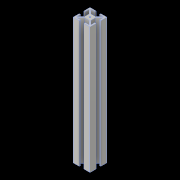
# Autodesk Inventor part: ProfileOne
Saved by Autodesk Inventor 2016 (Build 200138000, 138)
## iProperties
Created: 2017-01-21
Part Number: ProfileOne
Material: Generic
Document SubType Name: Modeling
Designer: Alexis Renderos
Density: 1 g/cm^3
Appearance: Aluminum - Flat
Author: Alexis Renderos
Autodesk Inventor part; units mm, degrees
ref_plane "YZ Plane" through (0, 0, 0) normal (1, 0, 0) x (0, 1, 0)
ref_plane "XZ Plane" through (0, 0, 0) normal (0, 1, 0) x (-1, 0, 0)
ref_plane "XY Plane" through (0, 0, 0) normal (0, 0, 1) x (1, 0, 0)
sketch "Sketch1" plane through (0, 0, 0) normal (0, 1, 0) x (-1, 0, 0)
  line L0 (0, -21.336) -> (0, 21.336) projected
  line L1 (-21.336, 0) -> (21.336, 0) projected
  line L2 (15.24, -15.24) -> (4.191, -15.24)
  line L3 (-15.24, -15.24) -> (-4.191, -15.24)
  line L4 (15.24, 4.191) -> (12.827, 4.191)
  line L5 (12.827, -4.191) -> (15.24, -4.191)
  line L6 (-4.191, 12.827) -> (-4.191, 15.24)
  line L7 (4.191, 15.24) -> (4.191, 12.827)
  line L8 (-11.1208, -12.827) -> (-4.212, -5.9182)
  line L9 (-12.827, -11.1208) -> (-5.9182, -4.212)
  line L10 (-5.9182, 4.212) -> (-12.827, 11.1208)
  line L11 (-4.212, 5.9182) -> (-11.1208, 12.827)
  line L12 (-1.7062, 0) -> (0, 1.7062)
  line L13 (4.212, 5.9182) -> (11.1208, 12.827)
  line L14 (0, -1.7062) -> (1.7062, 0)
  line L15 (5.9182, 4.212) -> (12.827, 11.1208)
  line L16 (12.827, -11.1208) -> (5.9182, -4.212)
  line L17 (1.7062, 0) -> (0, 1.7062)
  line L18 (11.1208, -12.827) -> (4.212, -5.9182)
  line L19 (0, -1.7062) -> (-1.7062, 0)
  line L20 (4.191, -12.827) -> (4.191, -15.24)
  line L21 (-15.24, 4.191) -> (-12.827, 4.191)
  line L22 (-4.191, -15.24) -> (-4.191, -12.827)
  line L23 (-12.827, -4.191) -> (-15.24, -4.191)
  line L24 (11.1208, 12.827) -> (4.191, 12.827)
  line L25 (-4.191, 12.827) -> (-11.1208, 12.827)
  line L26 (-12.827, 11.1208) -> (-12.827, 4.191)
  line L27 (-12.827, -4.191) -> (-12.827, -11.1208)
  line L28 (-11.1208, -12.827) -> (-4.191, -12.827)
  line L29 (4.191, -12.827) -> (11.1208, -12.827)
  line L30 (12.827, -11.1208) -> (12.827, -4.191)
  line L31 (12.827, 4.191) -> (12.827, 11.1208)
  line L32 (-15.24, -15.24) -> (-15.24, -4.191)
  line L33 (-15.24, 4.191) -> (-15.24, 15.24)
  line L34 (15.24, -15.24) -> (4.191, -15.24)
  line L35 (-4.191, -15.24) -> (-15.24, -15.24)
  line L36 (15.24, 15.24) -> (15.24, 4.191)
  line L37 (15.24, -4.191) -> (15.24, -15.24)
  line L38 (-15.24, 15.24) -> (-4.191, 15.24)
  line L39 (4.191, 15.24) -> (15.24, 15.24)
  line L40 (4.212, 5.9182) -> (-4.212, 5.9182)
  line L41 (-5.9182, 4.212) -> (-5.9182, -4.212)
  line L42 (-4.212, -5.9182) -> (4.212, -5.9182)
  line L43 (5.9182, -4.212) -> (5.9182, 4.212)
  line L44 (5.9182, 5.9182) -> (-5.9182, -5.9182) construction
  line L45 (-5.9182, 5.9182) -> (5.9182, -5.9182) construction
  point P0 (0, 0)
  point P1 (0, -4.191)
  point P2 (-4.191, 0)
  point P3 (0, 4.191)
  point P4 (4.191, 0)
  dimension "d4" = 11.049
  dimension "d5" = 30.48
  dimension "d6" = 30.48
  dimension "d15" = 11.8364
  dimension "d16" = 11.8364
  constraints: 88 end point, 22 parallel, 9 perpendicular, 8 point on line, 4 horizontal, 2 midpoint, 1 collinear
  measures "d4" distance of L3.end L3.start
  measures "d5" distance of L32.start L33.end
  measures "d6" distance of L33.end L36.start
  measures "d15" distance of L45.end L44.end
  measures "d16" distance of L44.end L45.start
extrude "Extrusion1" add sketch "Sketch1" along normal blind 228.6 contours L42 L8 L28 L22 L3 L32 L23 L27 L9 L41 L1 L19 L0 | L0 L14 L1 L43 L16 L30 L5 L37 L2 L20 L29 L18 L42 | L17 L0 L40 L13 L24 L7 L39 L36 L4 L31 L15 L43 L1 | L1 L41 L10 L26 L21 L33 L38 L6 L25 L11 L40 L0 L12
body "Solid1"
